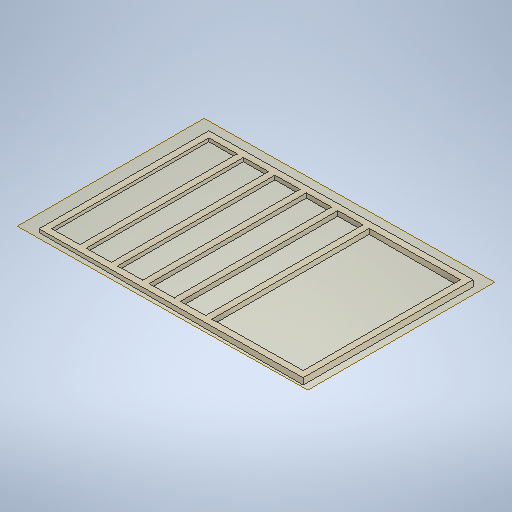
# Autodesk Inventor part: wing0.3.0
Saved by Autodesk Inventor 2025 (Build 290162000, 162)
## iProperties
Created: 2026-07-23
Part Number: wing0.3.0
Material: Generic
Document SubType Name: Modeling
Designer: DSTJOHN
Density: 1 g/cm^3
Appearance: Default
Author: DSTJOHN
Autodesk Inventor part; units mm, degrees
ref_plane "YZ Plane" through (0, 0, 0) normal (1, 0, 0) x (0, 1, 0)
ref_plane "XZ Plane" through (0, 0, 0) normal (0, 1, 0) x (-1, 0, 0)
ref_plane "XY Plane" through (0, 0, 0) normal (0, 0, 1) x (1, 0, 0)
sketch "Sketch1" plane through (0, 0, 0) normal (0, 1, 0) x (-1, 0, 0)
  line L0 (0, 0) -> (-84, 0)
  line L1 (-84, 0) -> (-84, -54)
  line L2 (-84, -54) -> (0, -54)
  line L3 (0, -54) -> (0, 0)
  line L4 (0, 0) -> (0, -2) construction
  line L5 (0, -2) -> (-2, -2) construction
  line L6 (-82, -2) -> (-82, -52)
  line L7 (-2, -52) -> (-2, -2)
  line L8 (-2, -52) -> (-11, -52) construction
  line L9 (-11, -2) -> (-11, -2)
  line L10 (-11, -52) -> (-11, -52)
  line L11 (-13, -2) -> (-13, -52)
  line L12 (-11, -52) -> (-11, -2)
  line L13 (-23, -2) -> (-23, -52)
  line L14 (-21, -52) -> (-21, -2)
  line L15 (-33, -2) -> (-33, -52)
  line L16 (-31, -52) -> (-31, -2)
  line L17 (-43, -2) -> (-43, -52)
  line L18 (-41, -52) -> (-41, -2)
  line L19 (-53, -2) -> (-53, -52)
  line L20 (-51, -52) -> (-51, -2)
  line L21 (-2, -2) -> (-11, -2)
  line L22 (-13, -2) -> (-21, -2)
  line L23 (-23, -2) -> (-31, -2)
  line L24 (-33, -2) -> (-41, -2)
  line L25 (-43, -2) -> (-51, -2)
  line L26 (-53, -2) -> (-82, -2)
  line L27 (-82, -52) -> (-53, -52)
  line L28 (-51, -52) -> (-43, -52)
  line L29 (-41, -52) -> (-33, -52)
  line L30 (-31, -52) -> (-23, -52)
  line L31 (-21, -52) -> (-13, -52)
  line L32 (-11, -52) -> (-2, -52)
  dimension "d0" = 84
  dimension "d1" = 54
  dimension "d3" = 2
  dimension "d4" = 80
  dimension "d5" = 50
  dimension "d7" = 2
  dimension "d8" = 9
  dimension "d9" = 2
  dimension "d10" = 19
  dimension "d11" = 2
  dimension "d12" = 29
  dimension "d14" = 2
  dimension "d15" = 39
  dimension "d16" = 2
  dimension "d17" = 49
  constraints: 66 end point, 45 parallel, 8 horizontal, 8 perpendicular, 2 point on line
  measures "d0" distance of L2.end L1.end
  measures "d1" distance of L1.end L0.end
  measures "d3" distance of L4.end L5.end
  measures "d4" distance of L7.start L6.end
  measures "d5" distance of L6.end L6.start
  measures "d7" distance between parallel lines of L11 L12
  measures "d8" distance between parallel lines of L12 L7
  measures "d9" distance between parallel lines of L13 L14
  measures "d10" distance between parallel lines of L14 L7
  measures "d11" distance between parallel lines of L15 L16
  measures "d12" distance between parallel lines of L7 L16
  measures "d14" distance between parallel lines of L17 L18
  measures "d15" distance between parallel lines of L18 L7
  measures "d16" distance between parallel lines of L19 L20
  measures "d17" distance between parallel lines of L20 L7
extrude "Extrusion1" add sketch "Sketch1" along normal blind 2
ref_plane "Work Plane1" through (84, 2, 0) normal (-0.0117, 0.9999, 0) x (0, 0, -1)
sketch "Sketch2" plane through (84, 2, 0) normal (-0.0117, 0.9999, 0) x (0, 0, -1)
  line L0 (56, 88) -> (-2, 88)
  line L1 (-2, 88) -> (-2, -3)
  line L2 (-2, -3) -> (56, -3)
  line L3 (56, -3) -> (56, 88)
  point P0 (0, 84.0176)
  constraints: 8 end point, 2 parallel, 1 horizontal, 1 perpendicular
extrude "Extrusion2" cut sketch "Sketch2" along normal blind 5.5
body "Solid1"
